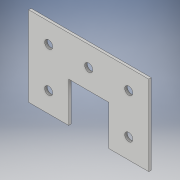
# Autodesk Inventor part: C-Bracket
Saved by Autodesk Inventor 2018 (Build 220112000, 112)
## iProperties
Created: 2019-01-15
Part Number: C-Bracket
Material: Generic
Document SubType Name: Modeling
Designer: maste
Density: 1 g/cm^3
Appearance: Default
Author: maste
Autodesk Inventor part; units mm, degrees
ref_plane "YZ Plane" through (0, 0, 0) normal (1, 0, 0) x (0, 1, 0)
ref_plane "XZ Plane" through (0, 0, 0) normal (0, 1, 0) x (-1, 0, 0)
ref_plane "XY Plane" through (0, 0, 0) normal (0, 0, 1) x (1, 0, 0)
sketch "Sketch1" plane through (0, 0, 0) normal (0, 0, 1) x (1, 0, 0)
  line L0 (0, 0) -> (25.4, 0)
  line L1 (25.4, 0) -> (25.4, 25.4)
  line L2 (25.4, 50.8) -> (0, 50.8)
  line L3 (0, 50.8) -> (0, 0)
  line L4 (0, 25.4) -> (0, 50.8)
  line L5 (12.7, 0) -> (12.7, 12.7) construction
  line L6 (12.7, 12.7) -> (12.7, 38.1) construction
  line L7 (12.7, 38.1) -> (38.1, 38.1) construction
  circle A0 centre (12.7, 12.7) radius 2.5797
  circle A1 centre (12.7, 38.1) radius 2.5797
  circle A2 centre (38.1, 38.1) radius 2.5797
  line L8 (25.4, 25.4) -> (50.8, 25.4)
  line L9 (50.8, 25.4) -> (50.8, 0)
  line L10 (50.8, 0) -> (76.2, 0)
  line L11 (76.2, 0) -> (76.2, 50.8)
  line L12 (76.2, 50.8) -> (25.4, 50.8)
  line L13 (38.1, 38.1) -> (63.5, 38.1) construction
  line L14 (63.5, 38.1) -> (63.5, 12.7) construction
  circle A3 centre (63.5, 38.1) radius 2.5797
  circle A4 centre (63.5, 12.7) radius 2.5797
  dimension "d0" = 25.4
  dimension "d1" = 50.8
  dimension "d5" = 12.7
  dimension "d6" = 25.4
  dimension "d7" = 25.4
  dimension "d11" = 5.1594
  dimension "d14" = 25.4
  dimension "d15" = 25.4
  dimension "d16" = 25.4
  dimension "d17" = 25.4
  constraints: 30 end point, 7 perpendicular, 5 centre point, 5 coincident, 3 horizontal, 2 parallel, 2 point on line, 1 midpoint, 1 vertical
  measures "d0" distance of L2.end L2.start
  measures "d1" distance of L2.start L0.end
  measures "d5" distance of L5.start L5.end
  measures "d6" distance of L5.end L6.end
  measures "d7" distance of L6.end L7.end
  measures "d11" diameter of A0
  measures "d14" distance of L1.end L8.end
  measures "d15" distance of L9.end L10.end
  measures "d16" distance of L13.start L13.end
  measures "d17" distance of L13.end L14.end
extrude "Extrusion2" add sketch "Sketch1" along normal blind 1.5875
body "Solid2"
